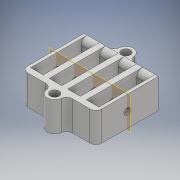
# Autodesk Inventor part: pulleyBottom
Saved by Autodesk Inventor 2018 (Build 220112000, 112)
## iProperties
Created: 2017-12-31
Part Number: pulleyBottom
Material: Generic
Document SubType Name: Modeling
Designer: mzhang
Density: 1 g/cm^3
Appearance: Default
Author: mzhang
Autodesk Inventor part; units mm, degrees
ref_plane "YZ Plane" through (0, 0, 0) normal (1, 0, 0) x (0, 1, 0)
ref_plane "XZ Plane" through (0, 0, 0) normal (0, 1, 0) x (-1, 0, 0)
ref_plane "XY Plane" through (0, 0, 0) normal (0, 0, 1) x (1, 0, 0)
sketch "Sketch1" plane through (0, 0, 0) normal (0, 0, 1) x (1, 0, 0)
  line L0 (0, 0) -> (4.25, 0)
  line L1 (4.25, 0) -> (4.25, 17)
  line L2 (4.25, 17) -> (0, 17)
  line L3 (0, 17) -> (0, 0)
  line L4 (-2, 19) -> (6.25, 19)
  line L5 (6.25, 19) -> (6.25, -2)
  line L6 (6.25, -2) -> (-2, -2)
  line L7 (-2, -2) -> (-2, 19)
  line L8 (5.25, 19) -> (5.25, -2)
  line L9 (-1, 19) -> (-1, -2)
  line L10 (5.25, 19) -> (5.25, -2)
  line L11 (4.25, 19) -> (12.5, 19)
  line L12 (11.5, 19) -> (11.5, -2)
  line L13 (12.5, -2) -> (4.25, -2)
  line L14 (10.5, 0) -> (10.5, 17)
  line L15 (6.25, 0) -> (10.5, 0)
  line L16 (6.25, 17) -> (6.25, 0)
  line L17 (11.5, 19) -> (11.5, -2)
  line L18 (10.5, 19) -> (18.75, 19)
  line L19 (17.75, 19) -> (17.75, -2)
  line L20 (18.75, -2) -> (10.5, -2)
  line L21 (16.75, 0) -> (16.75, 17)
  line L22 (12.5, 0) -> (16.75, 0)
  line L23 (12.5, 17) -> (12.5, 0)
  line L24 (17.75, 19) -> (17.75, -2)
  line L25 (16.75, 19) -> (25, 19)
  line L26 (24, 19) -> (24, -2)
  line L27 (25, -2) -> (16.75, -2)
  line L28 (23, 0) -> (23, 17)
  line L29 (18.75, 0) -> (23, 0)
  line L30 (18.75, 17) -> (18.75, 0)
  line L31 (10.5, 17) -> (6.25, 17)
  line L32 (12.5, 17) -> (16.75, 17)
  line L33 (18.75, 17) -> (23, 17)
  dimension "d0" = 4.25
  dimension "d1" = 17
  dimension "d2" = 2
  dimension "d5" = 6.25
  constraints: 68 end point, 16 point on line, 5 equal length, 5 perpendicular, 3 horizontal, 1 collinear, 59 other
  measures "d0" distance of L2.end L1.end
  measures "d1" distance of L0.end L1.end
  measures "d2" distance between parallel lines of L2 L4
  measures "d5" distance of L9.start L10.start
extrude "Extrusion1" add sketch "Sketch1" along normal blind 10 contours L4 L8 L6 L9 | L4 L5 L6 L8 | L11 L12 L13 L5 L15 L14 L31 | L11 L18 L19 L20 L13 L12 | L18 L25 L26 L27 L20 L19
sketch "Sketch2" plane through (24, -2, 0) normal (1, 0, 0) x (0, 0, -1)
  line L0 (0, 21) -> (-10, 21) projected
  line L1 (-10, 19) -> (-10, 2) projected
  point P0 (0, 2)
  point P1 (-5, 21)
  point P2 (-10, 10.5)
  point P3 (-5, 10.5)
  constraints: 2 midpoint
hole "Hole1" at (24, 8.5, 5) direction (-1, 0, 0) diameter 2.2 end through all
fillet "Fillet1" radius 2 8 edges at (2.125, 17, 10) (8.375, 17, 10) (14.625, 17, 10) (20.875, 17, 10) (20.875, 17, 0) (14.625, 17, 0) (8.375, 17, 0) (2.125, 17, 0)
fillet "Fillet2" radius 2 2 edges at (24, -2, 5) (-1, -2, 5)
sketch "Sketch3" plane through (0, 0, 10) normal (0, 0, 1) x (1, 0, 0)
  circle A0 centre (11.5859, -3.5) radius 1.5
  arc A1 (9.5859, -2) -> (13.5859, -2) centre (11.5859, -3.5) ccw
  line L0 (1, -2) -> (22, -2) projected
  point P0 (0, 0)
  dimension "d21" = 3
  dimension "d22" = 5
  dimension "d23" = 1.5
  constraints: 2 centre point, 2 point on circle, 2 point on line, 1 coincident
  measures "d21" diameter of A0
  measures "d22" diameter of A1
  measures "d23" distance from line of L0 A0.centre
extrude "Extrusion2" add sketch "Sketch3" against normal up to surface (10 mm away)
fillet "Fillet3" radius 2 2 edges at (9.5859, -2, 5) (13.5859, -2, 5)
ref_plane "Work Plane1" through (1, 8.5, 0) normal (0, -1, 0) x (1, 0, 0)
mirror "Mirror1" about plane through (1, 8.5, 0) normal (0, -1, 0) of "Extrusion2"
fillet "Fillet4" radius 2 2 edges at (13.5859, 19, 5) (9.5859, 19, 5)
chamfer "Chamfer1" distance 1 angle 30 8 edges at (4.25, 9.5, 0) (0, 9.5, 0) (6.25, 9.5, 0) (10.5, 9.5, 0) (12.5, 9.5, 0) (16.75, 9.5, 0) (18.75, 9.5, 0) (23, 9.5, 0) measured on face at (17.25, 9.5, 0) measured on face at (18.25, 9.5, 0) measured on face at (11, 9.5, 0) measured on face at (4.75, 9.5, 0) measured on face at (23.5, 9.5, 0) measured on face at (12, 9.5, 0) measured on face at (-0.5, 9.5, 0) measured on face at (5.75, 9.5, 0)
body "Solid1"
